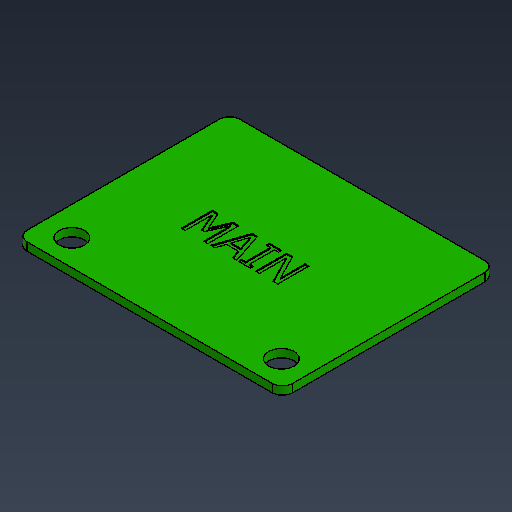
# Autodesk Inventor part: PCB_Controller
Saved by Autodesk Inventor 2026.2 (Build 302298010, 298A)
## iProperties
Created: 2026-04-05
Part Number: PCB_Controller
Material: Generic
Document SubType Name: Modeling
Designer: szymo
Density: 1 g/cm^3
Appearance: Default(1)
Author: szymo
Autodesk Inventor part; units mm, degrees
ref_plane "YZ Plane" through (0, 0, 0) normal (1, 0, 0) x (0, 1, 0)
ref_plane "XZ Plane" through (0, 0, 0) normal (0, 1, 0) x (-1, 0, 0)
ref_plane "XY Plane" through (0, 0, 0) normal (0, 0, 1) x (1, 0, 0)
ref_plane "Work Plane1" through (0.75, 0, 0.1) normal (0, 0, 1) x (1, 0, 0)
sketch "Sketch1" plane through (0.75, 0, 0.1) normal (0, 0, 1) x (1, 0, 0)
  circle A0 centre (15.45, 1.024) radius 2.1 projected
  circle A1 centre (15.45, -5.524) radius 2.1 projected
  line L0 (17.65, 4.2979) -> (17.65, -8.7979) projected
  line L1 (17.65, 4.2979) -> (13.85, 4.2979) projected
  line L2 (14.25, -8.7979) -> (14.25, -8.1479) projected
  line L3 (-17.65, 4.2979) -> (-17.65, -8.7979) projected
  line L4 (-17.65, -8.7979) -> (-13.25, -8.7979) projected
  line L5 (13.05, -5.9521) -> (-13.05, -5.9521)
  line L6 (-13.05, -5.9521) -> (-13.05, -5.1521)
  line L7 (-13.05, -5.1521) -> (13.05, -5.1521)
  line L8 (13.05, -5.1521) -> (13.05, -5.9521)
  line L9 (-13.25, 3.6479) -> (-13.25, -8.7979) projected
  circle A2 centre (-15.45, -5.524) radius 2.1 projected
  circle A3 centre (-15.45, 1.024) radius 2.1 projected
  line L10 (-14.25, 3.6479) -> (-13.25, 3.6479) projected
  line L11 (-14.25, 4.2979) -> (-14.25, 3.6479) projected
  line L12 (-17.65, 4.2979) -> (-14.25, 4.2979) projected
  line L13 (17.65, -8.7979) -> (14.25, -8.7979) projected
  line L14 (13.85, 3.6479) -> (13.85, 4.2979) projected
  line L15 (13.85, 3.6479) -> (13.25, 3.6479) projected
  line L16 (13.25, -8.1479) -> (13.25, 3.6479) projected
  line L17 (14.25, -8.1479) -> (13.25, -8.1479) projected
  point P0 (-0.75, 0)
  point P1 (13.65, 3.6479)
  dimension "d2" = 0.8
  dimension "d14" = 0.2
  dimension "d15" = 0.2
  constraints: 8 end point, 2 parallel, 1 horizontal, 1 perpendicular, 1 other
  measures "d2" distance between parallel lines of L7 L5
  measures "d14" distance between parallel lines of L16 L8
extrude "Extrusion1" add sketch "Sketch1" along normal blind 20.9 contours L5 L6 L7 L8
sketch "Sketch2" plane through (-12.3, -5.1521, 0.1) normal (0, 1, 0) x (1, 0, 0)
  line L0 (7.1098, -9.115) -> (17.2171, -9.115) construction
  line L1 (17.2171, -9.115) -> (17.2171, -12.163) construction
  line L2 (17.2171, -12.163) -> (7.1098, -12.163) construction
  line L3 (7.1098, -12.163) -> (7.1098, -9.115) construction
  line L4 (10.0318, -12.163) -> (9.6267, -12.163)
  line L5 (9.6267, -12.163) -> (9.6267, -9.5373)
  line L6 (9.6267, -9.5373) -> (8.8314, -11.3232)
  line L7 (8.8314, -11.3232) -> (8.5844, -11.3232)
  line L8 (8.5844, -11.3232) -> (7.7964, -9.5373)
  line L9 (7.7964, -9.5373) -> (7.7964, -12.163)
  line L10 (7.7964, -12.163) -> (7.4185, -12.163)
  line L11 (7.4185, -12.163) -> (7.4185, -9.115)
  line L12 (7.4185, -9.115) -> (7.9718, -9.115)
  line L13 (7.9718, -9.115) -> (8.7326, -10.8119)
  line L14 (8.7326, -10.8119) -> (9.4686, -9.115)
  line L15 (9.4686, -9.115) -> (10.0318, -9.115)
  line L16 (10.0318, -9.115) -> (10.0318, -12.163)
  line L17 (10.3208, -12.163) -> (11.3483, -9.115)
  line L18 (11.3483, -9.115) -> (11.8473, -9.115)
  line L19 (11.8473, -9.115) -> (12.8748, -12.163)
  line L20 (12.8748, -12.163) -> (12.4475, -12.163)
  line L21 (12.4475, -12.163) -> (12.1708, -11.3108)
  line L22 (12.1708, -11.3108) -> (11.0075, -11.3108)
  line L23 (11.0075, -11.3108) -> (10.7308, -12.163)
  line L24 (10.7308, -12.163) -> (10.3208, -12.163)
  line L25 (12.0597, -10.965) -> (11.5879, -9.5299)
  line L26 (11.5879, -9.5299) -> (11.1186, -10.965)
  line L27 (11.1186, -10.965) -> (12.0597, -10.965)
  line L28 (14.2259, -12.163) -> (13.0452, -12.163)
  line L29 (13.0452, -12.163) -> (13.0452, -11.8517)
  line L30 (13.0452, -11.8517) -> (13.433, -11.8517)
  line L31 (13.433, -11.8517) -> (13.433, -9.4262)
  line L32 (13.433, -9.4262) -> (13.0452, -9.4262)
  line L33 (13.0452, -9.4262) -> (13.0452, -9.115)
  line L34 (13.0452, -9.115) -> (14.2259, -9.115)
  line L35 (14.2259, -9.115) -> (14.2259, -9.4262)
  line L36 (14.2259, -9.4262) -> (13.8381, -9.4262)
  line L37 (13.8381, -9.4262) -> (13.8381, -11.8517)
  line L38 (13.8381, -11.8517) -> (14.2259, -11.8517)
  line L39 (14.2259, -11.8517) -> (14.2259, -12.163)
  line L40 (16.9083, -12.163) -> (16.4538, -12.163)
  line L41 (16.4538, -12.163) -> (15.1052, -9.5349)
  line L42 (15.1052, -9.5349) -> (15.1052, -12.163)
  line L43 (15.1052, -12.163) -> (14.7273, -12.163)
  line L44 (14.7273, -12.163) -> (14.7273, -9.115)
  line L45 (14.7273, -9.115) -> (15.3028, -9.115)
  line L46 (15.3028, -9.115) -> (16.5304, -11.5282)
  line L47 (16.5304, -11.5282) -> (16.5304, -9.115)
  line L48 (16.5304, -9.115) -> (16.9083, -9.115)
  line L49 (16.9083, -9.115) -> (16.9083, -12.163)
  point P0 (12.3, 0.1)
  dimension "d2" = 0.8
  dimension "d14" = 0.2
  dimension "d15" = 0.2
  constraints: 2 other
extrude "Extrusion2" cut sketch "Sketch2" against normal blind 0.1
sketch "Sketch3" plane through (-12.3, -5.9521, 0.1) normal (0, -1, 0) x (1, 0, 0)
  arc A0 (20.7, 16.6) -> (21.7, 15.6) centre (21.7, 16.6) ccw projected
  line L0 (26.2, 15.6) -> (21.7, 15.6) projected
  line L1 (26.2, 21.1) -> (26.2, 15.6) projected
  line L2 (20.7, 21.1) -> (26.2, 21.1) projected
  line L3 (20.7, 21.1) -> (20.7, 16.6) projected
  circle A1 centre (23.45, 18.35) radius 1.25 projected
  arc A2 (4.6, 15.6) -> (5.6, 16.6) centre (4.6, 16.6) ccw projected
  line L4 (5.6, 21.1) -> (5.6, 16.6) projected
  line L5 (0.1, 21.1) -> (5.6, 21.1) projected
  line L6 (0.1, 21.1) -> (0.1, 15.6) projected
  line L7 (4.6, 15.6) -> (0.1, 15.6) projected
  circle A3 centre (2.85, 18.35) radius 1.25 projected
  point P0 (12.3, -0.1)
  point P1 (22.45, 18.35)
  point P2 (2.55, 18.35)
hole "Hole1" at (11.15, -5.9521, 18.45) at (-9.45, -5.9521, 18.45) direction (0, 1, 0) diameter 2.5 end through all
fillet "Fillet1" radius 1 4 edges at (13.8, -5.5521, 0.1) (-12.3, -5.5521, 0.1) (-12.3, -5.5521, 21) (13.8, -5.5521, 21)
equation "\"d15\" = d14"
body "Solid1"
